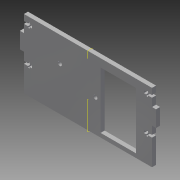
# Autodesk Inventor part: projectorMountingBase_RB01
Saved by Autodesk Inventor 2013 (Build 170138000, 138)
## iProperties
Created: 2014-06-13
Part Number: projectorMountingBase_RB01
Material: Steel, Wrought
Document SubType Name: Modeling
Designer: Byron
Density: 7.85 g/cm^3
Mass: 821.548 g
Surface Area: 397.604 cm^2
Volume: 104.656 cm^3
Author: Byron
Autodesk Inventor part; units mm, degrees
ref_plane "YZ Plane" through (0, 0, 0) normal (1, 0, 0) x (0, 1, 0)
ref_plane "XZ Plane" through (0, 0, 0) normal (0, 1, 0) x (-1, 0, 0)
ref_plane "XY Plane" through (0, 0, 0) normal (0, 0, 1) x (1, 0, 0)
sketch "Sketch1" plane through (0, 0, 0) normal (0, 0, 1) x (1, 0, 0)
  circle A0 centre (-45.2437, 35.97) radius 3.175
  circle A1 centre (10.6363, 18.2563) radius 3.175
  line L0 (-71.7503, -2.6941) -> (-71.7503, 45.5566)
  line L1 (69.7183, -2.6941) -> (-71.7503, -2.6941)
  line L2 (69.7183, 45.5566) -> (69.7183, -2.6941)
  line L3 (-71.7503, 45.5566) -> (69.7183, 45.5566)
  line L4 (99.568, 75.4063) -> (99.568, -32.5437)
  line L5 (99.568, -32.5437) -> (-101.6, -32.5438)
  line L6 (-101.6, -32.5438) -> (-101.6, 75.4062)
  line L7 (-101.6, 75.4062) -> (99.568, 75.4063)
  line L8 (18.8383, 62.7063) -> (74.667, 62.7063)
  line L9 (74.667, 62.7063) -> (74.667, -26.1937)
  line L10 (74.667, -26.1937) -> (18.8383, -26.1937)
  line L11 (18.8383, -26.1937) -> (18.8383, 62.7063)
  line L12 (99.568, 21.4313) -> (-101.6, 21.4312) construction
  line L13 (8.6043, 3.175) -> (8.6043, 21.4313) construction
  point P0 (0, 0)
  dimension "d2" = 201.168
  dimension "d3" = 107.95
  dimension "d4" = 107.95
  dimension "d5" = 90
  dimension "d6" = 201.168
  dimension "d7" = 12.7
  dimension "d8" = 88.9
  dimension "d26" = 39.4363
  dimension "d27" = 56.3563
  dimension "d28" = 6.35
  constraints: 28 end point, 2 centre point, 2 midpoint, 2 parallel, 2 perpendicular, 1 horizontal, 1 point on line, 3 other
  measures "d2" distance of L6.end L4.start
  measures "d3" distance of L4.start L4.end
  measures "d4" distance of L5.end L6.end
  measures "d5" angle of L5 L6
  measures "d6" distance of L4.end L5.end
  measures "d7" distance between parallel lines of L8 L7
  measures "d8" distance of L8.end L9.end
  measures "d26" distance from line of L7 A0.centre
  measures "d27" distance from line of L6 A0.centre
  measures "d28" diameter of A0
extrude "Extrusion1" add sketch "Sketch1" along normal blind 6.35 contours L0 L3 L11 L1 | L4 L5 L6 L7
sketch "Sketch2" plane through (0, 0, 0) normal (0, 0, -1) x (-1, 0, 0)
  line L0 (101.6, -32.5438) -> (101.6, 75.4062) projected
  line L1 (107.95, 65.692) -> (107.95, 61.9836) projected
  line L2 (107.95, 11.4304) -> (107.95, 7.722) projected
  line L3 (101.6, 7.722) -> (107.95, 7.722) construction
  line L4 (101.6, 11.4304) -> (107.95, 11.4304) construction
  line L5 (101.6, 61.9836) -> (107.95, 61.9836) construction
  line L6 (101.6, 65.4439) -> (107.95, 65.4439) construction
  line L7 (101.6, 7.722) -> (88.9, 7.722)
  line L8 (88.9, 7.722) -> (88.9, 11.4304)
  line L9 (88.9, 11.4304) -> (101.6, 11.4304)
  line L10 (101.6, 11.4304) -> (101.6, 7.722)
  line L11 (101.6, 61.9836) -> (88.9, 61.9836)
  line L12 (88.9, 61.9836) -> (88.9, 65.692)
  line L13 (88.9, 65.692) -> (101.6, 65.692)
  line L14 (101.6, 65.692) -> (101.6, 61.9836)
  line L15 (92.456, 5.6392) -> (95.25, 5.6392)
  line L16 (95.25, 5.6392) -> (95.25, 13.5132)
  line L17 (95.25, 13.5132) -> (92.456, 13.5132)
  line L18 (92.456, 13.5132) -> (92.456, 5.6392)
  line L19 (92.456, 59.9008) -> (95.25, 59.9008)
  line L20 (95.25, 59.9008) -> (95.25, 67.7748)
  line L21 (95.25, 67.7748) -> (92.456, 67.7748)
  line L22 (92.456, 67.7748) -> (92.456, 59.9008)
  point P0 (0, 0)
  dimension "d9" = 12.7
  dimension "d10" = 2.794
  dimension "d11" = 7.874
  dimension "d12" = 7.874
  dimension "d13" = 2.794
  dimension "d14" = 2.0828
  dimension "d16" = 2.0828
  dimension "d17" = 2.0828
  dimension "d18" = 6.35
  dimension "d19" = 6.35
  constraints: 40 end point, 12 horizontal, 8 parallel, 4 perpendicular, 5 other
  measures "d9" distance of L8.end L9.end
  measures "d10" distance of L17.end L16.end
  measures "d11" distance of L16.end L15.end
  measures "d12" distance of L20.end L19.end
  measures "d13" distance of L19.start L19.end
  measures "d14" distance between parallel lines of L15 L7
  measures "d16" distance between parallel lines of L17 L9
  measures "d17" distance between parallel lines of L19 L11
  measures "d18" distance between parallel lines of L0 L16
  measures "d19" distance between parallel lines of L0 L20
extrude "Extrusion2" cut sketch "Sketch2" against normal through all
ref_plane "Work Plane1" through (-1.016, -32.5437, 0) normal (-1, 0, 0) x (0, 0, 1)
mirror "Mirror1" about plane through (-1.016, -32.5437, 0) normal (-1, 0, 0) of "Extrusion2"
sketch "Sketch3" plane through (-101.6, 11.4304, 0) normal (-1, 0, 0) x (0, 0, 1)
  line L0 (0, 0) -> (0, 50.5532) projected
  line L1 (6.35, 0) -> (6.35, 50.5532) projected
  line L2 (6.35, 12.5766) -> (0, 12.5766) projected
  line L3 (0, 37.9766) -> (6.35, 37.9766) projected
  point P0 (0, -11.4304)
extrude "Extrusion3" add sketch "Sketch3" along normal blind 6.35
ref_plane "Work Plane2" through (-1.016, 75.4062, 6.35) normal (1, 0, 0) x (0, 0, -1)
mirror "Mirror2" about plane through (-1.016, 75.4062, 6.35) normal (1, 0, 0) of "Extrusion3"
equation "\"d4\" = d3"
equation "\"d6\" = d2"
equation "\"d13\" = d10"
equation "\"d14\" = d16"
equation "\"d17\" = d14"
equation "\"d19\" = d18"
body "Solid1"
